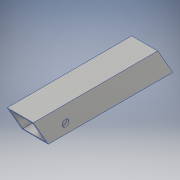
# Autodesk Inventor part: SUP_022_NEWClimberSupport
Saved by Autodesk Inventor 2018.3 (Build 223284000, 284)
## iProperties
Created: 2020-02-16
Part Number: SUP_022_NEWClimberSupport
Material: Aluminum 6061
Document SubType Name: Modeling
Designer: 22turnmaxw
Density: 2.7 g/cm^3
Appearance: Aluminum - Flat
Mass: 49.3935 g
Surface Area: 233.966 cm^2
Volume: 18.2939 cm^3
Author: 22turnmaxw
Autodesk Inventor part; units mm, degrees
ref_plane "YZ Plane" through (0, 0, 0) normal (1, 0, 0) x (0, 1, 0)
ref_plane "XZ Plane" through (0, 0, 0) normal (0, 1, 0) x (-1, 0, 0)
ref_plane "XY Plane" through (0, 0, 0) normal (0, 0, 1) x (1, 0, 0)
sketch "Sketch1" plane through (0, 0, 0) normal (0, 0, 1) x (1, 0, 0)
  line L0 (0, 0) -> (25.4, 0)
  line L1 (25.4, 0) -> (25.4, 25.4)
  line L2 (25.4, 25.4) -> (0, 25.4)
  line L3 (0, 25.4) -> (0, 0)
  line L4 (1.5875, 23.8125) -> (23.8125, 23.8125)
  line L5 (23.8125, 23.8125) -> (23.8125, 1.5875)
  line L6 (23.8125, 1.5875) -> (1.5875, 1.5875)
  line L7 (1.5875, 1.5875) -> (1.5875, 23.8125)
  dimension "d0" = 25.4
  dimension "d1" = 25.4
  dimension "d2" = 1.5875
  constraints: 16 end point, 4 parallel, 2 perpendicular, 1 horizontal, 3 other
  measures "d0" distance of L1.end L2.end
  measures "d1" distance of L2.end L0.start
  measures "d2" distance between parallel lines of L4 L2
extrude "Extrusion1" add sketch "Sketch1" along normal blind 203.2
sketch "Sketch3" plane through (25.4, 0, 0) normal (1, 0, 0) x (0, 0, -1)
  line L0 (0, 0) -> (-203.2, 0) projected
  line L1 (0, 0) -> (-14.6647, 25.4)
  line L2 (-14.6647, 25.4) -> (0, 25.4)
  line L3 (0, 23.8125) -> (-203.2, 23.8125) projected
  line L4 (0, 0) -> (0, 25.4) projected
  line L5 (0, 25.4) -> (0, 0)
  line L6 (0, 25.4) -> (-203.2, 25.4) projected
  line L7 (-192.6047, 25.4) -> (-177.94, 0)
  line L8 (0, 25.4) -> (-203.2, 25.4) projected
  line L9 (-192.6047, 25.4) -> (-203.2, 25.4)
  line L10 (-203.2, 25.4) -> (-203.2, 0)
  line L11 (-177.94, 0) -> (-203.2, 0)
  dimension "d8" = 30
  dimension "d11" = 177.94
  constraints: 14 end point, 3 collinear, 2 parallel, 2 perpendicular, 2 point on line
  measures "d8" angle of L4 L1
  measures "d11" distance of L0.start L7.end
extrude "Extrusion3" cut sketch "Sketch3" against normal blind 25.4 contours L1 L3 L4 | L1 L2 L4 L3
sketch "Sketch4" plane through (25.4, 0, 203.2) normal (1, 0, 0) x (0, 0, -1)
  line L0 (14.0789, 25.4) -> (28.7436, 0)
  line L1 (28.7436, 0) -> (0, 0)
  line L2 (189.4518, 23.8125) -> (0, 23.8125) projected
  line L3 (0, 0) -> (0, 25.4)
  line L4 (0, 25.4) -> (14.0789, 25.4)
  line L5 (188.5353, 25.4) -> (0, 25.4) projected
  line L6 (203.2, 0) -> (188.5353, 25.4) projected
  dimension "d12" = 174.4564
  dimension "d13" = 25.4
  dimension "d14" = 28.7436
  constraints: 8 end point, 2 collinear, 2 parallel, 1 perpendicular
  measures "d12" distance of L6.start L0.end
  measures "d13" distance of L1.end L3.end
  measures "d14" distance of L0.end L1.end
extrude "Extrusion4" cut sketch "Sketch4" against normal blind 25.4 contours L0 L2 L3 L4 | L0 L1 L3 L2
sketch "Sketch5" plane through (25.4, 0, 174.4564) normal (1, 0, 0) x (0, 0, -1)
  line L0 (173.5398, 1.5875) -> (-0.9165, 1.5875) projected
  line L1 (173.5398, 1.5875) -> (82.802, -50.8)
  line L2 (174.4564, 0) -> (159.7917, 25.4) projected
  line L3 (82.802, -50.8) -> (32.002, 37.1882)
  line L4 (159.7917, 25.4) -> (-14.6647, 25.4) projected
  line L5 (38.8079, 25.4) -> (-14.6647, 25.4)
  line L6 (-14.6647, 25.4) -> (0, 0)
  line L7 (0, 0) -> (53.4726, 0)
  line L8 (-14.6647, 25.4) -> (0, 0) projected
  line L9 (174.4564, 0) -> (0, 0) projected
  dimension "d17" = 90
  dimension "d18" = 104.775
  dimension "d20" = 101.6
  constraints: 10 end point, 3 collinear, 3 point on line, 1 parallel, 1 perpendicular
  measures "d17" angle of L1 L2
  measures "d18" distance of L0.start L1.end
  measures "d20" distance of L1.end L3.end
sketch "Sketch6" plane through (25.4, 0, 174.4564) normal (1, 0, 0) x (0, 0, -1)
  line L0 (159.7917, 25.4) -> (-14.6647, 25.4) projected
  line L1 (38.8079, 25.4) -> (53.4726, 0)
  line L2 (53.4726, 0) -> (0, 0)
  line L3 (173.5398, 1.5875) -> (-0.9165, 1.5875) projected
  line L4 (0, 0) -> (-14.6647, 25.4) projected
  line L5 (0, 0) -> (-14.6647, 25.4)
  line L6 (-14.6647, 25.4) -> (38.8079, 25.4)
  line L7 (160.7082, 23.8125) -> (-13.7482, 23.8125) projected
  line L8 (174.4564, 0) -> (0, 0) projected
  line L9 (82.802, -50.8) -> (32.002, 37.1882) projected
  constraints: 8 end point, 3 collinear, 2 parallel, 1 point on line
extrude "Extrusion5" cut sketch "Sketch6" against normal blind 25.4
sketch "Sketch7" plane through (25.4, 0, 120.9837) normal (1, 0, 0) x (0, 0, -1)
  line L0 (106.3191, 25.4) -> (-14.6647, 25.4) projected
  line L1 (-14.6647, 25.4) -> (29.3294, 50.8)
  line L2 (-14.6647, 25.4) -> (0, 0) projected
  line L3 (16.4978, 9.525) -> (16.4978, 9.525)
  line L4 (16.4978, 9.525) -> (0, 0)
  point P0 (120.9837, 0)
  dimension "d23" = 50.8
  dimension "d25" = 19.05
  dimension "d27" = 0
  constraints: 6 end point, 2 perpendicular, 1 parallel
  measures "d23" distance of L0.end L1.end
  measures "d25" distance of L3.end L2.end
  measures "d27" distance of L3.start L3.end
hole "Hole1" at (25.4, 9.525, 104.486) direction (-1, 0, 0) diameter 6.35 end through all
body "Solid1"
